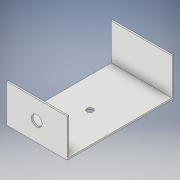
# Autodesk Inventor part: MAN_SERVO_HANDLER
Saved by Autodesk Inventor 2019 (Build 230136000, 136)
## iProperties
Created: 2021-03-07
Part Number: MAN_SERVO_HANDLER
Material: ABS Plastic
Document SubType Name: Modeling
Designer: DOMEK
Density: 1.06 g/cm^3
Appearance: Smooth - White
Author: DOMEK
Autodesk Inventor part; units mm, degrees
ref_plane "YZ Plane" through (0, 0, 0) normal (1, 0, 0) x (0, 1, 0)
ref_plane "XZ Plane" through (0, 0, 0) normal (0, 1, 0) x (-1, 0, 0)
ref_plane "XY Plane" through (0, 0, 0) normal (0, 0, 1) x (1, 0, 0)
sketch "Sketch6" plane through (0, 0, 0) normal (0, 1, 0) x (-1, 0, 0)
  line L0 (0, 0) -> (40, 0)
  line L1 (40, 0) -> (40, 70)
  line L2 (40, 70) -> (0, 70)
  line L3 (0, 70) -> (0, 0)
  dimension "d10" = 40
  dimension "d11" = 70
  constraints: 8 end point, 2 parallel, 1 horizontal, 1 perpendicular
  measures "d10" distance of L2.end L1.end
  measures "d11" distance of L1.end L0.end
extrude "Extrusion3" add sketch "Sketch6" along normal blind 25
shell "Shell1" thickness 1 removed faces 3 at (0, 8.3333, 46.6667) at (-40, 8.3333, 23.3333) at (-26.6667, 25, 23.3333)
sketch "Sketch7" plane through (-40, 0, 70) normal (0, 0, 1) x (1, 0, 0)
  line L0 (0, 25) -> (0, 1) projected
  line L1 (40, 0) -> (0, 0) projected
  line L2 (40, 1) -> (40, 25) projected
  circle A0 centre (20, 12.5) radius 3.5
  dimension "d15" = 7
  constraints: 1 centre point
  measures "d15" diameter of A0
extrude "Extrusion4" cut sketch "Sketch7" against normal blind 1
sketch "Sketch8" plane through (0, 0, 0) normal (0, -1, 0) x (1, 0, 0)
  line L0 (-40, 70) -> (0, 70) projected
  line L1 (0, 0) -> (-40, 0) projected
  circle A0 centre (-20, 35) radius 2
  dimension "d18" = 4
  constraints: 1 centre point
  measures "d18" diameter of A0
extrude "Extrusion5" cut sketch "Sketch8" against normal blind 1
body "Solid2"
